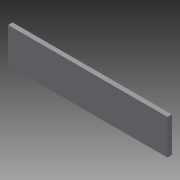
# Autodesk Inventor part: supportbeam1
Saved by Autodesk Inventor 2016 (Build 200138000, 138)
## iProperties
Created: 2016-01-29
Part Number: supportbeam1
Material: Generic
Document SubType Name: Modeling
Designer: zachary
Density: 1 g/cm^3
Appearance: Default
Mass: 9.26893 g
Surface Area: 67.2983 cm^2
Volume: 9.26893 cm^3
Author: zachary
Autodesk Inventor part; units mm, degrees
ref_plane "YZ Plane" through (0, 0, 0) normal (1, 0, 0) x (0, 1, 0)
ref_plane "XZ Plane" through (0, 0, 0) normal (0, 1, 0) x (-1, 0, 0)
ref_plane "XY Plane" through (0, 0, 0) normal (0, 0, 1) x (1, 0, 0)
sketch "Sketch1" plane through (0, 0, 0) normal (0, 0, 1) x (1, 0, 0)
  line L0 (0, 0) -> (-114.935, 0)
  line L1 (-114.935, 0) -> (-114.935, -25.4)
  line L2 (-114.935, -25.4) -> (0, -25.4)
  line L3 (0, -25.4) -> (0, 0)
  dimension "d0" = 25.4
  dimension "d1" = 114.935
  constraints: 8 end point, 2 parallel, 1 horizontal, 1 perpendicular
  measures "d0" distance between parallel lines of L0 L2
  measures "d1" distance between parallel lines of L1 L3
extrude "Extrusion1" add sketch "Sketch1" along normal blind 3.175
body "Solid1"
